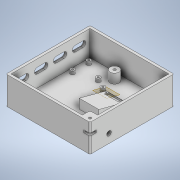
# Autodesk Inventor part: Caixa
Saved by Autodesk Inventor 2022 (Build 260153000, 153)
## iProperties
Created: 2022-03-20
Part Number: Caixa
Material: Genérico
Document SubType Name: Modeling
Designer: Hanter
Density: 1 g/cm^3
Appearance: Padrão
Author: Hanter
Autodesk Inventor part; units mm, degrees
ref_plane "YZ Plane" through (0, 0, 0) normal (1, 0, 0) x (0, 1, 0)
ref_plane "XZ Plane" through (0, 0, 0) normal (0, 1, 0) x (-1, 0, 0)
ref_plane "XY Plane" through (0, 0, 0) normal (0, 0, 1) x (1, 0, 0)
sketch "Esboço1" plane through (0, 0, 0) normal (0, 1, 0) x (-1, 0, 0)
  line L0 (-62.5, 62.5) -> (62.5, 62.5)
  line L1 (62.5, 62.5) -> (62.5, -62.5)
  line L2 (62.5, -62.5) -> (-62.5, -62.5)
  line L3 (-62.5, -62.5) -> (-62.5, 62.5)
  line L4 (-62.5, 62.5) -> (62.5, -62.5) construction
  line L5 (62.5, 62.5) -> (-62.5, -62.5) construction
  point P0 (0, 0)
  dimension "d0" = 125
  dimension "d1" = 125
  constraints: 12 end point, 2 midpoint, 2 parallel, 1 horizontal, 1 perpendicular
  measures "d0" distance of L0.start L0.end
  measures "d1" distance of L2.end L0.start
extrude "Extrusão1" add sketch "Esboço1" along normal blind 4
sketch "Esboço2" plane through (0, 4, 0) normal (0, 1, 0) x (1, 0, 0)
  line L0 (-57.5, 55.5) -> (-21.5, 55.5)
  line L1 (-21.5, 55.5) -> (-21.5, 34.5)
  line L2 (-21.5, 34.5) -> (-57.5, 34.5)
  line L3 (-57.5, 34.5) -> (-57.5, 55.5)
  line L4 (62.5, 62.5) -> (-62.5, 62.5) projected
  line L5 (-62.5, 62.5) -> (-62.5, -62.5) projected
  circle A0 centre (-55, 53) radius 1.4
  circle A1 centre (-24, 37) radius 1.4
  circle A2 centre (-55, 53) radius 3.5
  circle A3 centre (-24, 37) radius 3.5
  line L6 (-57.6, 29.9977) -> (-4.6, 29.9977)
  line L7 (-4.6, 29.9977) -> (-4.6, -40.0023)
  line L8 (-4.6, -40.0023) -> (-57.6, -40.0023)
  line L9 (-57.6, -40.0023) -> (-57.6, 29.9977)
  circle A4 centre (-55.1, 27.4977) radius 1.45
  circle A5 centre (-55.1, -37.5023) radius 1.45
  circle A6 centre (-7.1, -37.5023) radius 1.45
  circle A7 centre (-7.1, 27.4977) radius 1.45
  circle A8 centre (-55.1, 27.4977) radius 3.5
  circle A9 centre (-7.1, 27.4977) radius 3.5
  circle A10 centre (-7.1, -37.5023) radius 3.5
  circle A11 centre (-55.1, -37.5023) radius 3.5
  line L10 (-1, 31) -> (27, 59) construction
  line L11 (27, 31) -> (-1, 59) construction
  line L12 (56, 55.5) -> (35, 55.5)
  line L13 (35, 55.5) -> (35, 12.5)
  line L14 (35, 12.5) -> (56, 12.5)
  line L15 (56, 12.5) -> (56, 55.5)
  circle A12 centre (53.5, 49) radius 1.4
  circle A13 centre (37.5, 19) radius 1.4
  line L16 (62.5, -62.5) -> (62.5, 62.5) projected
  circle A14 centre (53.5, 49) radius 3.5
  circle A15 centre (37.5, 19) radius 3.5
  line L17 (-62.5, -62.5) -> (62.5, -62.5) projected
  circle A16 centre (-11.5, 50.5) radius 2
  circle A17 centre (-11.5, 50.5) radius 3.5
  line L18 (-11.5, 54.6208) -> (-7.9313, 52.5604)
  line L19 (-7.9313, 52.5604) -> (-7.9313, 48.4396)
  line L20 (-7.9313, 48.4396) -> (-11.5, 46.3792)
  line L21 (-11.5, 46.3792) -> (-15.0687, 48.4396)
  line L22 (-15.0687, 48.4396) -> (-15.0687, 52.5604)
  line L23 (-15.0687, 52.5604) -> (-11.5, 54.6208)
  point P0 (0, 0)
  point P1 (13, 45)
  dimension "d7" = 5
  dimension "d9" = 2.8
  dimension "d10" = 2.5
  dimension "d11" = 2.5
  dimension "d12" = 2.5
  dimension "d13" = 2.5
  dimension "d14" = 7
  dimension "d15" = 7
  dimension "d16" = 53
  dimension "d17" = 70
  dimension "d18" = 2.9
  dimension "d19" = 2.9
  dimension "d20" = 2.9
  dimension "d21" = 2.9
  dimension "d22" = 48
  dimension "d23" = 2.5
  dimension "d25" = 48
  dimension "d26" = 2.5
  dimension "d27" = 65
  dimension "d28" = 2.5
  dimension "d29" = 7
  dimension "d30" = 7
  dimension "d31" = 7
  dimension "d32" = 7
  dimension "d39" = 21
  dimension "d40" = 43
  dimension "d41" = 2.8
  dimension "d42" = 2.8
  dimension "d43" = 7
  dimension "d44" = 6.5
  dimension "d45" = 6.5
  dimension "d46" = 2.5
  dimension "d47" = 6.5
  dimension "d48" = 2.5
  dimension "d49" = 7
  dimension "d50" = 7
  dimension "d51" = 2.8
  dimension "d57" = 36
  dimension "d58" = 21
  dimension "d83" = 22.4977
  dimension "d160" = 4
  dimension "d161" = 12
  dimension "d162" = 51
  dimension "d163" = 7
  constraints: 40 end point, 18 centre point, 10 coincident, 6 parallel, 3 horizontal, 3 perpendicular, 2 midpoint, 13 other
  measures "d7" distance between parallel lines of L5 L3
  measures "d9" diameter of A1
  measures "d10" distance from line of L0 A0.centre
  measures "d11" distance from line of L3 A0.centre
  measures "d12" distance from line of L1 A1.centre
  measures "d13" distance from line of L2 A1.centre
  measures "d14" diameter of A2
  measures "d15" diameter of A3
  measures "d16" distance of L7.end L8.end
  measures "d17" distance of L6.end L7.end
  measures "d18" diameter of A4
  measures "d19" diameter of A5
  measures "d20" diameter of A6
  measures "d21" diameter of A7
  measures "d22" distance of A6.centre A5.centre
  measures "d23" distance from line of L9 A5.centre
  measures "d25" distance of A7.centre A4.centre
  measures "d26" distance from line of L9 A4.centre
  measures "d27" distance of A4.centre A5.centre
  measures "d28" distance from line of L8 A5.centre
  measures "d29" diameter of A8
  measures "d30" diameter of A9
  measures "d31" diameter of A10
  measures "d32" diameter of A11
  measures "d39" distance of L14.end L13.end
  measures "d40" distance of L13.end L12.end
  measures "d41" diameter of A12
  measures "d42" diameter of A13
  measures "d43" distance between parallel lines of L12 L4
  measures "d44" distance between parallel lines of L16 L15
  measures "d45" distance from line of L12 A12.centre
  measures "d46" distance from line of L15 A12.centre
  measures "d47" distance from line of L14 A13.centre
  measures "d48" distance from line of L13 A13.centre
  measures "d49" diameter of A14
  measures "d50" diameter of A15
  measures "d51" diameter of A0
  measures "d57" distance of L0.start L0.end
  measures "d58" distance of L0.end L1.end
  measures "d83" distance between parallel lines of L17 L8
  measures "d160" diameter of A16
  measures "d161" distance from line of L4 A16.centre
  measures "d162" distance from line of L5 A16.centre
  measures "d163" diameter of A17
extrude "Extrusão2" add sketch "Esboço2" along normal blind 5 contours A2 L0 | L0 A2 L3 | L3 A2 | A3 L1 | L1 A3 L2 | L2 A3 | A8 L6 | L6 A8 L9 | L9 A8 | A9 L6 | L6 A9 L7 | A11 L8 L9 | L9 A11 | L7 A9 | A10 L7 | L7 A10 L8 | L8 A11 | L8 A10 | A14 L15 | L15 A14 | A15 L13 | L13 A15 picked at (-55.0563, 55.1299) picked at (-24.0563, 34.8701) picked at (-55.1583, 29.6442) picked at (-7.1583, 29.6442) picked at (-55.1583, -39.6488) picked at (-7.1583, -39.6488)
sketch "Esboço5" plane through (0, 9, 0) normal (0, 1, 0) x (1, 0, 0)
  circle A0 centre (29.5, 45) radius 1.45
  line L0 (29.5, 50) -> (27, 50) projected
  line L1 (25.5, 57.5) -> (25.5, 32.5) projected
  point P0 (0, 0)
  dimension "d70" = 2.9
  dimension "d71" = 5
  dimension "d72" = 4
  constraints: 1 centre point
  measures "d70" diameter of A0
  measures "d71" distance from line of L0 A0.centre
  measures "d72" distance from line of L1 A0.centre
extrude "Extrusão5" cut sketch "Esboço5" against normal blind 5
sketch "Esboço6" plane through (0, 4, 0) normal (0, 1, 0) x (1, 0, 0)
  line L0 (0, 26) -> (31, 26)
  line L1 (31, 26) -> (31, -17)
  line L2 (31, -17) -> (0, -17)
  line L3 (0, -17) -> (0, 26)
  line L4 (0, -17) -> (31, -17)
  line L5 (-1, 31) -> (27, 31) projected
  line L6 (-57.5, -40.0023) -> (-4.5, -40.0023)
  line L7 (-4.5, -40.0023) -> (-4.5, 29.9977)
  line L8 (-4.5, 29.9977) -> (-57.5, 29.9977)
  line L9 (-57.5, 29.9977) -> (-57.5, -40.0023)
  line L10 (-62.5, 62.5) -> (-62.5, -62.5) projected
  line L11 (-62.5, -62.5) -> (62.5, -62.5) projected
  line L12 (56, 12.5) -> (35, 12.5)
  line L13 (35, 12.5) -> (35, 55.5)
  line L14 (35, 55.5) -> (56, 55.5)
  line L15 (56, 55.5) -> (56, 12.5)
  line L16 (62.5, 62.5) -> (-62.5, 62.5) projected
  line L17 (62.5, -62.5) -> (62.5, 62.5) projected
  point P0 (0, 0)
  dimension "d76" = 43
  dimension "d78" = 5
  dimension "d79" = 53
  dimension "d80" = 70
  dimension "d81" = 5
  dimension "d82" = 22.4977
  dimension "d84" = 21
  dimension "d85" = 43
  dimension "d86" = 7
  dimension "d87" = 6.5
  dimension "d88" = 4.5
  constraints: 26 end point, 6 parallel, 4 horizontal, 3 perpendicular
  measures "d76" distance of L0.end L1.end
  measures "d78" distance between parallel lines of L5 L0
  measures "d79" distance of L8.end L7.end
  measures "d80" distance of L7.end L6.end
  measures "d81" distance between parallel lines of L10 L9
  measures "d82" distance between parallel lines of L11 L6
  measures "d84" distance of L13.end L14.end
  measures "d85" distance of L12.end L13.end
  measures "d86" distance between parallel lines of L16 L14
  measures "d87" distance between parallel lines of L17 L15
  measures "d88" distance between parallel lines of L7 L3
extrude "Extrusão6" add sketch "Esboço6" along normal blind 24 contours L0 L1 L2 L3
sketch "Esboço7" plane through (31, 4, 17) normal (1, 0, 0) x (0, 0, -1)
  line L0 (43.4351, 3.6251) -> (-38.6686, 25.6247)
  line L1 (-45.5, 0) -> (79.5, 0) projected
  line L2 (43.4351, 3.6251) -> (43.4351, 27.2402)
  line L3 (43.4351, 27.2402) -> (-38.6686, 25.6247)
  point P0 (17, -4)
  dimension "d92" = 85
  dimension "d93" = 15
  constraints: 6 end point, 1 vertical
  measures "d92" distance of L0.start L0.end
  measures "d93" angle of L1 L0
extrude "Extrusão7" cut sketch "Esboço7" against normal blind 31
sketch "Esboço8" plane through (0, 19.2634, 17) normal (0, 0.9659258, -0.258819) x (1, 0, 0)
  circle A0 centre (2.5, 41.5169) radius 0.95
  circle A1 centre (28.5, 41.5169) radius 0.95
  line L0 (0, 44.5169) -> (31, 44.5169) projected
  line L1 (0, 0) -> (0, 44.5169) projected
  line L2 (31, 44.5169) -> (31, 0) projected
  point P0 (0, 21.4065)
  dimension "d96" = 1.9
  dimension "d97" = 1.9
  dimension "d98" = 3
  dimension "d99" = 2.5
  dimension "d100" = 3
  dimension "d101" = 2.5
  constraints: 2 centre point
  measures "d96" diameter of A0
  measures "d97" diameter of A1
  measures "d98" distance from line of L0 A0.centre
  measures "d99" distance from line of L1 A0.centre
  measures "d100" distance from line of L0 A1.centre
  measures "d101" distance from line of L2 A1.centre
extrude "Extrusão8" cut sketch "Esboço8" against normal blind 4
ref_plane "Plano de trabalho2" through (2.5, 8.0976, -23.2575) normal (0, 0.9659258, -0.258819) x (1, 0, 0)
sketch "Esboço10" plane through (2.5, 8.0976, -23.2575) normal (0, 0.9659258, -0.258819) x (1, 0, 0)
  line L0 (2.2, -5.4) -> (23.8, -5.4)
  line L1 (23.8, -5.4) -> (23.8, 2.3)
  line L2 (23.8, 2.3) -> (2.2, 2.3)
  line L3 (2.2, 2.3) -> (2.2, -5.4)
  line L4 (-2.5, -41.5169) -> (-2.5, 3) projected
  line L5 (28.5, 3) -> (28.5, -41.5169) projected
  line L6 (-2.5, 3) -> (28.5, 3) projected
  point P0 (-2.5, -20.3692)
  dimension "d108" = 4.7
  dimension "d109" = 4.7
  dimension "d110" = 0.7
  dimension "d111" = 7.7
  constraints: 8 end point, 2 parallel, 1 horizontal, 1 perpendicular
  measures "d108" distance between parallel lines of L4 L3
  measures "d109" distance between parallel lines of L5 L1
  measures "d110" distance between parallel lines of L6 L2
  measures "d111" distance between parallel lines of L2 L0
extrude "Extrusão10" cut sketch "Esboço10" along normal mid plane 3.7
sketch "Esboço11" plane through (0, 0, 0) normal (0, -1, 0) x (1, 0, 0)
  line L0 (-66.5, -66.5) -> (66.5, -66.5)
  line L1 (66.5, -66.5) -> (66.5, 66.5)
  line L2 (66.5, 66.5) -> (-66.5, 66.5)
  line L3 (-66.5, 66.5) -> (-66.5, -66.5)
  line L4 (-66.5, -66.5) -> (66.5, 66.5) construction
  line L5 (66.5, -66.5) -> (-66.5, 66.5) construction
  line L6 (62.5, 62.5) -> (62.5, -62.5) projected
  line L7 (-62.5, -62.5) -> (62.5, -62.5)
  line L8 (62.5, -62.5) -> (62.5, 62.5)
  line L9 (62.5, 62.5) -> (-62.5, 62.5)
  line L10 (-62.5, 62.5) -> (-62.5, -62.5)
  line L11 (-62.5, -62.5) -> (62.5, 62.5) construction
  line L12 (62.5, -62.5) -> (-62.5, 62.5) construction
  point P0 (0, 0)
  dimension "d114" = 133
  dimension "d115" = 133
  constraints: 24 end point, 4 midpoint, 4 parallel, 2 horizontal, 2 perpendicular
  measures "d114" distance of L2.end L1.end
  measures "d115" distance of L1.end L0.end
extrude "Extrusão11" add sketch "Esboço11" against normal blind 44
fillet "Arredondamento2" radius 2 4 edges at (-66.5, 22, 66.5) (66.5, 22, 66.5) (66.5, 22, -66.5) (-66.5, 22, -66.5)
sketch "Esboço13" plane through (-66.5, 0, -64.5) normal (-1, 0, 0) x (0, 0, 1)
  arc A0 (13.41, 32.65) -> (13.41, 23.35) centre (13.41, 28) ccw
  line L0 (0, 44) -> (129, 44) projected
  arc A1 (25.41, 23.35) -> (25.41, 32.65) centre (25.41, 28) ccw
  line L1 (13.41, 32.65) -> (25.41, 32.65)
  line L2 (25.41, 23.35) -> (13.41, 23.35)
  arc A2 (43.47, 32.65) -> (43.47, 23.35) centre (43.47, 28) ccw
  arc A3 (55.47, 23.35) -> (55.47, 32.65) centre (55.47, 28) ccw
  line L3 (43.47, 32.65) -> (55.47, 32.65)
  line L4 (55.47, 23.35) -> (43.47, 23.35)
  arc A4 (73.53, 32.65) -> (73.53, 23.35) centre (73.53, 28) ccw
  arc A5 (85.53, 23.35) -> (85.53, 32.65) centre (85.53, 28) ccw
  line L5 (73.53, 32.65) -> (85.53, 32.65)
  line L6 (85.53, 23.35) -> (73.53, 23.35)
  arc A6 (103.59, 32.65) -> (103.59, 23.35) centre (103.59, 28) ccw
  arc A7 (115.59, 23.35) -> (115.59, 32.65) centre (115.59, 28) ccw
  line L7 (103.59, 32.65) -> (115.59, 32.65)
  line L8 (115.59, 23.35) -> (103.59, 23.35)
  line L9 (131, 0) -> (131, 44) projected
  line L10 (-2, 44) -> (-2, 0) projected
  line L11 (129, 44) -> (129, 0) projected
  line L12 (0, 0) -> (0, 44) projected
  point P0 (64.5, 0)
  dimension "d131" = 9.3
  dimension "d132" = 16
  dimension "d133" = 9.3
  dimension "d134" = 12
  dimension "d135" = 9.3
  dimension "d136" = 9.3
  dimension "d137" = 12
  dimension "d138" = 9.3
  dimension "d139" = 9.3
  dimension "d140" = 12
  dimension "d141" = 9.3
  dimension "d142" = 9.3
  dimension "d143" = 12
  dimension "d145" = 16
  dimension "d146" = 16
  dimension "d147" = 16
  dimension "d150" = 13.41
  dimension "d151" = 18.06
  dimension "d152" = 18.06
  dimension "d153" = 18.06
  constraints: 16 end point, 16 point on circle, 12 tangent, 8 centre point
  measures "d131" diameter of A0
  measures "d132" distance from line of L0 A0.centre
  measures "d133" diameter of A1
  measures "d134" distance of A1.centre A0.centre
  measures "d135" diameter of A2
  measures "d136" diameter of A3
  measures "d137" distance of A3.centre A2.centre
  measures "d138" diameter of A4
  measures "d139" diameter of A5
  measures "d140" distance of A5.centre A4.centre
  measures "d141" diameter of A6
  measures "d142" diameter of A7
  measures "d143" distance of A7.centre A6.centre
  measures "d145" distance from line of L0 A2.centre
  measures "d146" distance from line of L0 A4.centre
  measures "d147" distance from line of L0 A6.centre
  measures "d150" distance from line of L12 A0.centre
  measures "d151" distance of A1.centre A2.centre
  measures "d152" distance of A4.centre A3.centre
  measures "d153" distance of A6.centre A5.centre
extrude "Extrusão12" cut sketch "Esboço13" against normal blind 5
sketch "Esboço15" plane through (0, 44, 0) normal (0, 1, 0) x (1, 0, 0)
  circle A0 centre (-11.5, 50.5) radius 2
  line L0 (-62.5, 62.5) -> (62.5, 62.5) projected
  line L1 (-62.5, -62.5) -> (-62.5, 62.5) projected
  line L2 (-11.5, 54.7301) -> (-7.8366, 52.6151)
  line L3 (-7.8366, 52.6151) -> (-7.8366, 48.3849)
  line L4 (-7.8366, 48.3849) -> (-11.5, 46.2699)
  line L5 (-11.5, 46.2699) -> (-15.1634, 48.3849)
  line L6 (-15.1634, 48.3849) -> (-15.1634, 52.6151)
  line L7 (-15.1634, 52.6151) -> (-11.5, 54.7301)
  circle A1 centre (-11.5, 50.5) radius 7
  point P0 (0, 0)
  point P1 (56, 62.5)
  dimension "d164" = 4
  dimension "d165" = 12
  dimension "d166" = 51
  dimension "d168" = 14
  constraints: 12 end point, 2 centre point, 1 coincident, 13 other
  measures "d164" diameter of A0
  measures "d165" distance from line of L0 A0.centre
  measures "d166" distance from line of L1 A0.centre
  measures "d168" diameter of A1
extrude "Extrusão14" add sketch "Esboço15" against normal blind 40 contours A1
sketch "Esboço18" plane through (-62.5, 4, -62.5) normal (0, 0, 1) x (1, 0, 0)
  line L0 (125, 40) -> (0, 40) projected
  line L1 (43.5378, 40) -> (60.5378, 40)
  line L2 (60.5378, 40) -> (60.5378, 10)
  line L3 (60.5378, 10) -> (43.5378, 10)
  line L4 (43.5378, 10) -> (43.5378, 40)
  point P0 (62.5, -4)
  dimension "d179" = 30
  dimension "d182" = 17
  constraints: 8 end point, 2 parallel, 1 horizontal, 1 perpendicular, 1 point on line
  measures "d179" distance of L1.end L2.end
  measures "d182" distance between parallel lines of L4 L2
extrude "Extrusão16" cut sketch "Esboço18" along normal blind 20.7
sketch "Esboço19" plane through (0, 4, 0) normal (0, 1, 0) x (1, 0, 0)
  line L0 (-11.5, 54.7301) -> (-7.8366, 52.6151)
  line L1 (-7.8366, 52.6151) -> (-7.8366, 48.3849)
  line L2 (-7.8366, 48.3849) -> (-11.5, 46.2699)
  line L3 (-11.5, 46.2699) -> (-15.1634, 48.3849)
  line L4 (-15.1634, 48.3849) -> (-15.1634, 52.6151)
  line L5 (-15.1634, 52.6151) -> (-11.5, 54.7301)
  point P0 (0, 0)
  point P1 (-11.5, 50.5)
  constraints: 12 end point, 13 other
extrude "Extrusão17" add sketch "Esboço19" along normal blind 5.9
sketch "Esboço20" plane through (-11.5, 14, -50.5) normal (0, 1, 0) x (1, 0, 0)
  circle A0 centre (0, 0) radius 7
  point P0 (11.5, -50.5)
  constraints: 1 centre point
extrude "Extrusão18" add sketch "Esboço20" along normal blind 5
sketch "Esboço21" plane through (-11.5, 19, -50.5) normal (0, 1, 0) x (1, 0, 0)
  circle A0 centre (0, 0) radius 2
  point P0 (11.5, -50.5)
  dimension "d187" = 4
  constraints: 1 centre point
  measures "d187" diameter of A0
extrude "Extrusão19" cut sketch "Esboço21" against normal blind 16
sketch "Esboço22" plane through (0, 44, 0) normal (0, 1, 0) x (1, 0, 0)
  line L0 (-62.5, -62.5) -> (62.5, -62.5) projected
  line L1 (62.5, -62.5) -> (50.5, -62.5)
  line L2 (50.5, -62.5) -> (50.5, -50.5)
  line L3 (50.5, -50.5) -> (62.5, -50.5)
  line L4 (62.5, -50.5) -> (62.5, -62.5)
  point P0 (0, 0)
  dimension "d192" = 12
  dimension "d193" = 12
  constraints: 8 end point, 2 parallel, 1 horizontal, 1 perpendicular
  measures "d192" distance of L2.end L3.end
  measures "d193" distance of L1.end L2.end
extrude "Extrusão20" add sketch "Esboço22" against normal blind 40
fillet "Arredondamento3" radius 3 1 edges at (50.5, 24, 50.5)
sketch "Esboço24" plane through (-64.5, 0, 66.5) normal (0, 0, 1) x (1, 0, 0)
  line L0 (131, 44) -> (131, 0) projected
  line L1 (131, 29) -> (121, 29)
  line L2 (121, 29) -> (121, 25)
  line L3 (121, 25) -> (131, 25)
  line L4 (131, 25) -> (131, 29)
  line L5 (0, 44) -> (129, 44) projected
  point P0 (64.5, 0)
  dimension "d197" = 10
  dimension "d198" = 4
  dimension "d199" = 15
  constraints: 8 end point, 2 parallel, 1 horizontal, 1 perpendicular, 1 point on line
  measures "d197" distance of L3.end L2.end
  measures "d198" distance of L2.end L1.end
  measures "d199" distance between parallel lines of L5 L1
extrude "Extrusão21" cut sketch "Esboço24" against normal blind 10
sketch "Esboço25" plane through (0, 44, 0) normal (0, 1, 0) x (1, 0, 0)
  circle A0 centre (60.5, -60.5) radius 2.005
  line L0 (66.5, -64.5) -> (66.5, 64.5) projected
  line L1 (-64.5, -66.5) -> (64.5, -66.5) projected
  point P0 (0, 0)
  dimension "d202" = 4.01
  dimension "d203" = 6
  dimension "d204" = 6
  constraints: 1 centre point
  measures "d202" diameter of A0
  measures "d203" distance from line of L0 A0.centre
  measures "d204" distance from line of L1 A0.centre
extrude "Extrusão22" cut sketch "Esboço25" against normal blind 36.75
sketch "Esboço26" plane through (66.5, 0, 64.5) normal (1, 0, 0) x (0, 0, -1)
  circle A0 centre (28, 14) radius 3.6
  line L0 (129, 0) -> (0, 0) projected
  line L1 (-2, 25) -> (-2, 0) projected
  point P0 (64.5, 0)
  dimension "d207" = 7.2
  dimension "d208" = 14
  dimension "d209" = 30
  constraints: 1 centre point
  measures "d207" diameter of A0
  measures "d208" distance from line of L0 A0.centre
  measures "d209" distance from line of L1 A0.centre
extrude "Extrusão23" cut sketch "Esboço26" against normal blind 5
